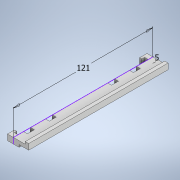
# Autodesk Inventor part: scratcher
Saved by Autodesk Inventor 2022 (Build 260153000, 153)
## iProperties
Created: 2023-01-26
Part Number: scratcher
Material: Generic
Document SubType Name: Modeling
Designer: CLCK
Density: 1 g/cm^3
Appearance: Default
Author: CLCK
Autodesk Inventor part; units mm, degrees
ref_plane "YZ Plane" through (0, 0, 0) normal (1, 0, 0) x (0, 1, 0)
ref_plane "XZ Plane" through (0, 0, 0) normal (0, 1, 0) x (-1, 0, 0)
ref_plane "XY Plane" through (0, 0, 0) normal (0, 0, 1) x (1, 0, 0)
sketch "Sketch1" plane through (0, 0, 0) normal (1, 0, 0) x (0, 1, 0)
  line L0 (4.9903, 57.7832) -> (9.9903, 57.7832)
  line L1 (9.9903, 57.7832) -> (9.9903, -63.2168)
  line L2 (9.9903, -63.2168) -> (4.9903, -63.2168)
  line L3 (4.9903, -63.2168) -> (4.9903, 57.7832)
  point P0 (0, 0)
  dimension "d0" = 121
  dimension "d1" = 5
  constraints: 8 end point, 2 parallel, 1 horizontal, 1 perpendicular
  measures "d0" distance of L0.end L1.end
  measures "d1" distance of L1.end L2.end
extrude "Extrusion1" add sketch "Sketch1" along normal blind 5
sketch "Sketch2" plane through (0, 0, 0) normal (-1, 0, 0) x (0, 0, 1)
  line L0 (-63.2168, 9.9903) -> (57.7832, 9.9903) projected
  line L1 (57.7832, 4.9903) -> (-63.2168, 4.9903) projected
  line L2 (57.7832, 9.9903) -> (53.7832, 9.9903)
  line L3 (53.7832, 9.9903) -> (53.7832, 4.9903)
  line L4 (53.7832, 4.9903) -> (57.7832, 4.9903)
  line L5 (57.7832, 4.9903) -> (57.7832, 9.9903)
  line L6 (-63.2168, 4.9903) -> (-63.2168, 9.9903) projected
  line L7 (-63.2168, 9.9903) -> (-59.2168, 9.9903)
  line L8 (-59.2168, 9.9903) -> (-59.2168, 4.9903)
  line L9 (-59.2168, 4.9903) -> (-63.2168, 4.9903)
  line L10 (-63.2168, 4.9903) -> (-63.2168, 9.9903)
  point P0 (0, 0)
  dimension "d4" = 4
  dimension "d5" = 4
  constraints: 16 end point, 4 parallel, 2 horizontal, 2 perpendicular, 2 point on line
  measures "d4" distance between parallel lines of L5 L3
  measures "d5" distance between parallel lines of L6 L8
extrude "Extrusion2" add sketch "Sketch2" along normal blind 5 contours L0 L8 L1 L6 | L0 L5 L1 L3
sketch "Sketch3" plane through (5, 9.9903, 57.7832) normal (0, 1, 0) x (1, 0, 0)
  line L0 (-10, 4) -> (-10, 0) projected
  line L1 (-10, 4) -> (-8, 4)
  line L2 (-8, 4) -> (-8, 6)
  line L3 (-8, 6) -> (-10, 6)
  line L4 (-10, 6) -> (-10, 4)
  line L5 (-10, 117) -> (-10, 121) projected
  line L6 (-10, 117) -> (-8, 117)
  line L7 (-8, 117) -> (-8, 114.6592)
  line L8 (-8, 114.6592) -> (-10, 114.6592)
  line L9 (-10, 114.6592) -> (-10, 117)
  point P0 (-5, 57.7832)
  dimension "d8" = 2
  dimension "d9" = 2
  constraints: 16 end point, 4 parallel, 2 horizontal, 2 perpendicular, 1 point on line
  measures "d8" distance of L3.end L0.start
  measures "d9" distance of L2.end L3.end
extrude "Extrusion3" add sketch "Sketch3" against normal blind 5
sketch "Sketch4" plane through (5, 4.9903, -63.2168) normal (0, 0, -1) x (-1, 0, 0)
  line L0 (10, 5) -> (0, 5) projected
  line L1 (0, 5) -> (-5.3853, 5)
  line L2 (-5.3853, 5) -> (-5.3853, 7)
  line L3 (-5.3853, 7) -> (-8.3853, 7)
  line L4 (-8.3853, 7) -> (-8.3853, 2)
  line L5 (-8.3853, 2) -> (0, 2)
  line L6 (0, 0) -> (0, 5) projected
  line L7 (0, 5) -> (0, 2)
  point P0 (5, -4.9903)
  dimension "d12" = 3
  dimension "d13" = 3
  dimension "d14" = 2
  dimension "d15" = 5
  constraints: 12 end point, 1 collinear, 1 horizontal
  measures "d12" distance between parallel lines of L5 L1
  measures "d13" distance of L2.end L3.end
  measures "d14" distance of L1.end L2.end
  measures "d15" distance of L3.end L4.end
extrude "Extrusion4" add sketch "Sketch4" against normal up to surface (121 mm away)
sketch "Sketch5" plane through (0, 9.9903, 53.7832) normal (0, 1, 0) x (1, 0, 0)
  line L0 (-4.4204, 23.7832) -> (3.5, 23.7832)
  line L1 (3.5, 23.7832) -> (3.5, 29.7832)
  line L2 (3.5, 29.7832) -> (-4.4204, 29.7832)
  line L3 (-4.4204, 29.7832) -> (-4.4204, 23.7832)
  line L4 (-4.4204, 77.7832) -> (3.5, 77.7832)
  line L5 (3.5, 77.7832) -> (3.5, 83.7832)
  line L6 (3.5, 83.7832) -> (-4.4204, 83.7832)
  line L7 (-4.4204, 83.7832) -> (-4.4204, 77.7832)
  line L8 (10.3853, 117) -> (10.3853, -4) projected
  line L9 (-4.4204, 4.7832) -> (3.5, 4.7832)
  line L10 (3.5, 4.7832) -> (3.5, 10.7832)
  line L11 (3.5, 10.7832) -> (-4.4204, 10.7832)
  line L12 (-4.4204, 10.7832) -> (-4.4204, 4.7832)
  line L13 (-4.4204, 96.7832) -> (3.5, 96.7832)
  line L14 (3.5, 96.7832) -> (3.5, 102.7832)
  line L15 (3.5, 102.7832) -> (-4.4204, 102.7832)
  line L16 (-4.4204, 102.7832) -> (-4.4204, 96.7832)
  line L17 (0, 113) -> (0, 0) projected
  point P0 (0, 53.7832)
  dimension "d18" = 6
  dimension "d20" = 6
  dimension "d21" = 24
  dimension "d22" = 24
  dimension "d25" = 6
  dimension "d26" = 6
  dimension "d27" = 43
  dimension "d28" = 43
  dimension "d31" = 3.5
  dimension "d32" = 3.5
  constraints: 32 end point, 8 parallel, 5 collinear, 4 horizontal, 4 perpendicular
  measures "d18" distance of L2.end L0.start
  measures "d20" distance of L6.end L4.start
  measures "d21" distance from line of L4 point (0, 53.783)
  measures "d22" distance from line of point (0, 53.783) L2
  measures "d25" distance of L11.end L9.start
  measures "d26" distance of L15.end L13.start
  measures "d27" distance from line of L13 point (0, 53.783)
  measures "d28" distance from line of L11 point (0, 53.783)
  measures "d31" distance between parallel lines of L5 L17
  measures "d32" distance between parallel lines of L17 L1
extrude "Extrusion5" cut sketch "Sketch5" against normal blind 10
body "Solid1"
